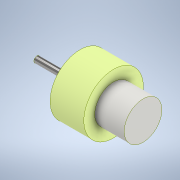
# Autodesk Inventor part: DC MOTOR NEW
Saved by Autodesk Inventor 2021 (Build 250183000, 183)
## iProperties
Created: 2021-07-10
Part Number: DC MOTOR NEW
Material: Generic
Document SubType Name: Modeling
Designer: HP
Density: 1 g/cm^3
Appearance: Zinc Chromate 2
Author: HP
Autodesk Inventor part; units mm, degrees
ref_plane "YZ Plane" through (0, 0, 0) normal (1, 0, 0) x (0, 1, 0)
ref_plane "XZ Plane" through (0, 0, 0) normal (0, 1, 0) x (-1, 0, 0)
ref_plane "XY Plane" through (0, 0, 0) normal (0, 0, 1) x (1, 0, 0)
sketch "Sketch1" plane through (0, 0, 0) normal (1, 0, 0) x (0, 1, 0)
  circle A0 centre (0, 0) radius 11.2253
  constraints: 1 centre point, 1 coincident
extrude "Extrusion1" add sketch "Sketch1" along normal blind 12.7
sketch "Sketch2" plane through (0, 0, 0) normal (-1, 0, 0) x (0, 0, 1)
  line L0 (-4.7625, 0) -> (-2.3813, 4.1244)
  line L1 (-2.3813, 4.1244) -> (2.3812, 4.1244)
  line L2 (2.3812, 4.1244) -> (4.7625, 0)
  line L3 (4.7625, 0) -> (2.3813, -4.1244)
  line L4 (2.3813, -4.1244) -> (-2.3812, -4.1244)
  line L5 (-2.3812, -4.1244) -> (-4.7625, 0)
  circle A0 centre (0, 0) radius 1.5875
  point P0 (1.6165, 3.316)
  constraints: 12 end point, 1 centre point, 1 coincident, 13 other
extrude "Extrusion2" add sketch "Sketch2" along normal blind 2.54
sketch "Sketch3" plane through (-2.54, 0, 0) normal (-1, 0, 0) x (0, 0, 1)
  circle A0 centre (0, 0) radius 1.143
  dimension "d4" = 2.286
  constraints: 1 centre point
  measures "d4" diameter of A0
extrude "Extrusion3" add sketch "Sketch3" along normal blind 13.6525 and the other way blind 8.4201
sketch "Sketch4" plane through (12.7, 0, 0) normal (1, 0, 0) x (0, 0, -1)
  circle A0 centre (0, 0) radius 7.0995
  constraints: 1 centre point, 1 coincident
extrude "Extrusion4" add sketch "Sketch4" along normal blind 11.1125
body "Solid1"
